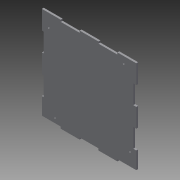
# Autodesk Inventor part: Side Panel
Saved by Autodesk Inventor 2015 SP1 (Build 190203100, 203)
## iProperties
Created: 2015-08-25
Part Number: Side Panel
Material: Generic
Document SubType Name: Modeling
Designer: Kartikye
Density: 1 g/cm^3
Appearance: Default
Author: Kartikye
Autodesk Inventor part; units mm, degrees
ref_plane "YZ Plane" through (0, 0, 0) normal (1, 0, 0) x (0, 1, 0)
ref_plane "XZ Plane" through (0, 0, 0) normal (0, 1, 0) x (-1, 0, 0)
ref_plane "XY Plane" through (0, 0, 0) normal (0, 0, 1) x (1, 0, 0)
sketch "Sketch1" plane through (0, 0, 0) normal (0, 1, 0) x (-1, 0, 0)
  line L0 (-25, -25) -> (25, -25)
  line L1 (25, -25) -> (25, 25)
  line L2 (25, 25) -> (-25, 25)
  line L3 (-25, 25) -> (-25, -25)
  line L4 (-25, -25) -> (25, 25) construction
  line L5 (25, -25) -> (-25, 25) construction
  point P0 (0, 0)
  dimension "d0" = 50
  dimension "d1" = 50
  constraints: 12 end point, 2 midpoint, 2 parallel, 1 horizontal, 1 perpendicular
  measures "d0" distance of L0.start L0.end
  measures "d1" distance of L1.end L0.end
extrude "Extrusion1" add sketch "Sketch1" along normal blind 1
sketch "Sketch2" plane through (0, 1, 0) normal (0, 1, 0) x (1, 0, 0)
  line L0 (25, -25) -> (25, -15)
  line L1 (25, -25) -> (25, 25) projected
  line L2 (25, -15) -> (23.4, -15)
  line L3 (23.4, -15) -> (23.4, -5)
  line L4 (23.4, -5) -> (25, -5)
  line L5 (25, -5) -> (25, 5)
  line L6 (25, 5) -> (23.4, 5)
  line L7 (23.4, 5) -> (23.4, 15)
  line L8 (23.4, 15) -> (25, 15)
  line L9 (25, 15) -> (25, 25)
  line L10 (27, 25) -> (27, -25)
  line L11 (27, -25) -> (25, -25)
  point P0 (0, 0)
  dimension "d4" = 1.6
  dimension "d5" = 10
  dimension "d6" = 10
  constraints: 22 end point, 6 point on line, 4 perpendicular, 1 collinear, 1 horizontal
  measures "d4" distance of L0.end L2.end
  measures "d5" distance of L2.end L3.end
  measures "d6" distance of L4.end L5.end
extrude "Extrusion2" cut sketch "Sketch2" against normal blind 1
sketch "Sketch3" plane through (0, 1, 0) normal (0, 1, 0) x (1, 0, 0)
  line L0 (25, 25) -> (25, 24)
  line L1 (25, 24) -> (15, 24)
  line L2 (15, 24) -> (15, 25)
  line L3 (25, 25) -> (-25, 25) projected
  line L4 (15, 25) -> (5, 25)
  line L5 (5, 25) -> (5, 24)
  line L6 (5, 24) -> (-5, 24)
  line L7 (-5, 24) -> (-5, 25)
  line L8 (-5, 25) -> (-15, 25)
  line L9 (-15, 25) -> (-15, 24)
  line L10 (-15, 24) -> (-25, 24)
  line L11 (-25, 24) -> (-25, 27)
  line L12 (-25, 27) -> (25, 27)
  line L13 (25, 27) -> (25, 25)
  point P0 (0, 0)
  constraints: 26 end point, 8 point on line, 5 perpendicular, 1 vertical
extrude "Extrusion3" cut sketch "Sketch3" against normal blind 1
sketch "Sketch4" plane through (0, 1, 0) normal (0, 1, 0) x (1, 0, 0)
  line L0 (-25, -25) -> (-25, -15)
  line L1 (-25, -15) -> (-24, -15)
  line L2 (-24, -15) -> (-24, -5)
  line L3 (-24, -5) -> (-25, -5)
  line L4 (-25, 24) -> (-25, -25) projected
  line L5 (-25, -5) -> (-25, 5)
  line L6 (-25, 24) -> (-25, -25) projected
  line L7 (-25, 5) -> (-24, 5)
  line L8 (-24, 5) -> (-24, 15)
  line L9 (-24, 15) -> (-25, 15)
  line L10 (-25, 24) -> (-27, 23)
  line L11 (-27, 23) -> (-27, -24.2648)
  line L12 (-27, -24.2648) -> (-25, -25)
  point P0 (0, 0)
  dimension "d11" = 10
  dimension "d12" = 10
  dimension "d13" = 10
  constraints: 22 end point, 5 point on line, 4 perpendicular, 1 vertical
  measures "d11" distance of L0.start L0.end
  measures "d12" distance of L3.end L5.end
  measures "d13" distance of L7.end L8.end
extrude "Extrusion4" cut sketch "Sketch4" against normal blind 1 contours L4 L3 L2 L1 | L4 L9 L8 L7
sketch "Sketch5" plane through (0, 1, 0) normal (0, 1, 0) x (1, 0, 0)
  line L0 (-25, -25) -> (-15, -25)
  line L1 (-25, -25) -> (25, -25) projected
  line L2 (-15, -25) -> (-15, -24)
  line L3 (-15, -24) -> (-5, -24)
  line L4 (-5, -24) -> (-5, -25)
  line L5 (-5, -25) -> (5, -25)
  line L6 (5, -25) -> (5, -24)
  line L7 (5, -24) -> (15, -24)
  line L8 (15, -24) -> (15, -25)
  line L9 (25, -25) -> (25, -26)
  line L10 (25, -26) -> (-25, -26)
  line L11 (-25, -26) -> (-25, -25)
  point P0 (0, 0)
  dimension "d16" = 10
  constraints: 22 end point, 5 perpendicular, 3 point on line
  measures "d16" distance of L0.start L0.end
extrude "Extrusion5" cut sketch "Sketch5" against normal blind 1 contours L2 L3 L4 L1 | L6 L7 L8 L1
sketch "Sketch6" plane through (0, 1, 0) normal (0, 1, 0) x (1, 0, 0)
  circle A0 centre (-21.5, -18.2) radius 0.5
  circle A1 centre (-18.2, 21.5) radius 0.5
  circle A2 centre (18.2, -21.5) radius 0.5
  circle A3 centre (21.5, 17.2) radius 0.5
  line L0 (15, -25) -> (25, -25) projected
  line L1 (25, -25) -> (25, -15) projected
  line L2 (-25, -25) -> (-15, -25) projected
  line L3 (-25, -15) -> (-25, -25) projected
  line L4 (-5, 25) -> (-15, 25) projected
  line L5 (-25, 24) -> (-25, 15) projected
  line L6 (25, 24) -> (15, 24) projected
  line L7 (25, 15) -> (25, 24) projected
  point P0 (0, 0)
  dimension "d21" = 1
  dimension "d22" = 1
  dimension "d23" = 1
  dimension "d24" = 1
  dimension "d25" = 3.5
  dimension "d26" = 6.8
  dimension "d27" = 6.8
  dimension "d28" = 3.5
  dimension "d29" = 3.5
  dimension "d30" = 6.8
  dimension "d31" = 6.8
  dimension "d32" = 3.5
  constraints: 4 centre point
  measures "d21" diameter of A0
  measures "d22" diameter of A1
  measures "d23" diameter of A2
  measures "d24" diameter of A3
  measures "d25" distance from line of L0 A2.centre
  measures "d26" distance from line of L1 A2.centre
  measures "d27" distance from line of L2 A0.centre
  measures "d28" distance from line of A0.centre L3
  measures "d29" distance from line of L4 A1.centre
  measures "d30" distance from line of L5 A1.centre
  measures "d31" distance from line of L6 A3.centre
  measures "d32" distance from line of L7 A3.centre
extrude "Extrusion6" cut sketch "Sketch6" against normal blind 1
body "Solid1"
